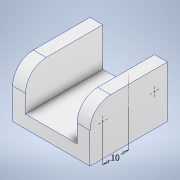
# Autodesk Inventor part: WheelArm
Saved by Autodesk Inventor 2020 (Build 240168000, 168)
## iProperties
Created: 2019-12-17
Part Number: WheelArm
Material: Aluminum 6061
Document SubType Name: Modeling
Designer: Kjell
Density: 2.7 g/cm^3
Appearance: Aluminum - Flat
Author: Kjell
Autodesk Inventor part; units mm, degrees
ref_plane "YZ Plane" through (0, 0, 0) normal (1, 0, 0) x (0, 1, 0)
ref_plane "XZ Plane" through (0, 0, 0) normal (0, 1, 0) x (-1, 0, 0)
ref_plane "XY Plane" through (0, 0, 0) normal (0, 0, 1) x (1, 0, 0)
sketch "Sketch1" plane through (0, 0, 0) normal (1, 0, 0) x (0, 1, 0)
  line L0 (-7, 7.5) -> (15, 7.5)
  line L1 (15, 7.5) -> (15, -7.5)
  line L2 (15, -7.5) -> (-15, -7.5)
  line L3 (-15, -7.5) -> (-15, -0.5)
  line L4 (-15, 7.5) -> (15, -7.5) construction
  line L5 (15, 7.5) -> (-15, -7.5) construction
  arc A0 (-7, 7.5) -> (-15, -0.5) centre (-7, -0.5) ccw
  point P0 (0, 0)
  dimension "d0" = 30
  dimension "d1" = 15
  dimension "d2" = 8
  constraints: 12 end point, 2 midpoint, 2 parallel, 2 point on circle, 2 point on line, 2 tangent, 1 centre point, 1 horizontal, 1 perpendicular
  measures "d0" distance of L1.end L2.end
  measures "d1" distance of L0.end L1.end
  measures "d2" radius of A0
extrude "Extrusion1" add sketch "Sketch1" along normal mid plane 30
sketch "Sketch2" plane through (15, 15, -7.5) normal (0, 0, -1) x (-1, 0, 0)
  line L0 (5, 0.0565) -> (25, 0.0565)
  line L1 (25, 0.0565) -> (25, -30)
  line L2 (25, -30) -> (5, -30)
  line L3 (5, -30) -> (5, 0.0565)
  line L4 (15, -15) -> (15, 7.3899) construction
  line L5 (0, -30) -> (0, 0) projected
  line L6 (30, -30) -> (0, -30) projected
  dimension "d5" = 5
  constraints: 10 end point, 2 parallel, 1 horizontal, 1 perpendicular, 1 vertical, 1 other
  measures "d5" distance between parallel lines of L3 L5
extrude "Extrusion2" cut sketch "Sketch2" against normal up to next
sketch "Sketch4" plane through (15, -15, -7.5) normal (0, 0, -1) x (-1, 0, 0)
  line L0 (0, 8) -> (0, 0) projected
  line L1 (25, 30) -> (30, 30) projected
  line L2 (0, 0) -> (30, 0)
  line L3 (30, 0) -> (30, 30)
  line L4 (30, 30) -> (0, 30)
  line L5 (0, 30) -> (0, 0)
  point P0 (15, 15)
  constraints: 8 end point, 2 parallel, 1 horizontal, 1 perpendicular
extrude "Extrusion4" add sketch "Sketch4" along normal blind 5
sketch "Sketch5" plane through (15, 0, 0) normal (1, 0, 0) x (0, 0, -1)
  line L0 (0, 0) -> (-10.8374, 0) construction
  point P0 (0, -10)
  point P1 (0, 10)
  dimension "d14" = 10
  constraints: 2 end point, 2 vertical alignment, 1 horizontal, 1 symmetric about line
  measures "d14" distance of L0.start point (0, -10)
sketch "Sketch6" plane through (-15, 0, 0) normal (-1, 0, 0) x (0, 0, 1)
  point P0 (0, 0)
  point P1 (0, -10)
  point P2 (0, 10)
sketch "Sketch3" plane through (-15, -15, -7.5) normal (0, -1, 0) x (1, 0, 0)
  line L0 (5, 5) -> (25, 5)
  line L1 (25, 5) -> (25, 16.3557)
  line L2 (25, 16.3557) -> (5, 16.3557)
  line L3 (5, 16.3557) -> (5, 5)
  line L4 (0, 0) -> (30, 0) projected
  line L5 (5, 15) -> (5, 7) projected
  line L6 (25, 7) -> (25, 15) projected
  point P0 (15, 7.5)
  point P1 (5, 11)
  point P2 (25, 11)
  dimension "d9" = 5
  constraints: 8 end point, 2 midpoint, 2 parallel, 2 point on line, 1 horizontal, 1 perpendicular
  measures "d9" distance between parallel lines of L4 L0
body "Solid1"
